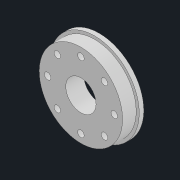
# Autodesk Inventor part: base9
Saved by Autodesk Inventor 2022 (Build 260153000, 153)
## iProperties
Created: 2021-09-17
Part Number: base9
Material: 一般
Document SubType Name: Modeling
Designer: Yuta Kage
Density: 1 g/cm^3
Appearance: 既定
Author: Yuta Kage
Autodesk Inventor part; units mm, degrees
ref_plane "YZ Plane" through (0, 0, 0) normal (1, 0, 0) x (0, 1, 0)
ref_plane "XZ Plane" through (0, 0, 0) normal (0, 1, 0) x (-1, 0, 0)
ref_plane "XY Plane" through (0, 0, 0) normal (0, 0, 1) x (1, 0, 0)
sketch "スケッチ1" plane through (0, 0, 0) normal (1, 0, 0) x (0, 1, 0)
  line L0 (10, 0) -> (27.5, 0)
  line L1 (27.5, 0) -> (27.5, -9)
  line L2 (27.5, -9) -> (29.5, -9)
  line L3 (29.5, -9) -> (29.5, -12)
  line L4 (10, -12) -> (10, 0)
  line L5 (0, -14.4) -> (0, 2.4) projected
  line L6 (29.5, -12) -> (10, -12)
  point P0 (0, 0)
  dimension "d5" = 9
  dimension "d30" = 2
  dimension "d31" = 27.5
  dimension "d32" = 3
  constraints: 12 end point, 4 perpendicular, 1 horizontal, 1 horizontal alignment
  measures "d5" distance of L0.end L1.end
  measures "d30" distance of L1.end L2.end
  measures "d31" distance between parallel lines of L5 L1
  measures "d32" distance of L2.end L3.end
revolve "回転1" add sketch "スケッチ1" angle 360 about axis through (0, 0, -10) along (0, 0, 1)
sketch "スケッチ2" plane through (0, 0, 0) normal (0, 0, 1) x (1, 0, 0)
  circle A0 centre (0, 0) radius 22
  point P0 (0, 22)
  point P1 (-15.5563, 15.5563)
  point P2 (-22, 0)
  point P3 (-15.5563, -15.5563)
  point P4 (0, -22)
  point P5 (15.5563, -15.5563)
  point P6 (22, 0)
  point P7 (15.5563, 15.5563)
  dimension "d11" = 44
  dimension "d14" = 360
  constraints: 1 coincident, 1 vertical alignment, 11 other
hole "穴1" at (0, 22, 0) at (-15.5563, 15.5563, 0) at (-22, 0, 0) at (-15.5563, -15.5563, 0) at (0, -22, 0) at (15.5563, -15.5563, 0) at (22, 0, 0) at (15.5563, 15.5563, 0) direction (0, 0, -1) diameter 4.3 end through all clearance for "Socket Head Cap Screw" size "M4" standard "Ansi Metric M Profile"
